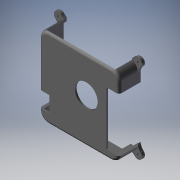
# Autodesk Inventor part: BP004
Saved by Autodesk Inventor 2017 SP1 (Build 210196100, 196)
## iProperties
Created: 2018-01-04
Part Number: BP004
Material: ABS Plastic
Document SubType Name: Modeling
Designer: Zach
Density: 1.06 g/cm^3
Appearance: CR White
Author: Zach
Autodesk Inventor part; units mm, degrees
ref_plane "YZ Plane" through (0, 0, 0) normal (1, 0, 0) x (0, 1, 0)
ref_plane "XZ Plane" through (0, 0, 0) normal (0, 1, 0) x (-1, 0, 0)
ref_plane "XY Plane" through (0, 0, 0) normal (0, 0, 1) x (1, 0, 0)
sketch "Sketch1" plane through (0, 0, 0) normal (0, 0, 1) x (1, 0, 0)
  line L0 (0, 0) -> (140, 0)
  line L1 (140, 0) -> (140, 140)
  line L2 (140, 140) -> (0, 140)
  line L3 (0, 140) -> (0, 0)
  line L4 (5, 135) -> (135, 135)
  line L5 (135, 135) -> (135, 5)
  line L6 (135, 5) -> (5, 5)
  line L7 (5, 5) -> (5, 135)
  point P0 (70, 135)
  point P1 (70, 140)
  point P2 (135, 70)
  point P3 (140, 70)
  dimension "d0" = 140
  dimension "d1" = 140
  dimension "d2" = 130
  dimension "d3" = 130
  constraints: 16 end point, 4 midpoint, 4 parallel, 2 horizontal, 2 perpendicular, 1 horizontal alignment, 1 vertical alignment
  measures "d0" distance of L2.end L1.end
  measures "d1" distance of L1.end L0.end
  measures "d2" distance of L5.end L6.end
  measures "d3" distance of L4.end L5.end
extrude "Extrusion1" add sketch "Sketch1" along normal blind 35
sketch "Sketch2" plane through (0, 0, 35) normal (0, 0, 1) x (1, 0, 0)
  line L0 (135, 5) -> (5, 5) projected
  line L1 (135, 135) -> (135, 5) projected
  line L2 (135, 5) -> (5, 5) projected
  line L3 (5, 5) -> (5, 135) projected
  line L4 (5, 135) -> (135, 135) projected
  line L5 (0, 0) -> (140, 0) projected
  line L6 (140, 0) -> (140, 140) projected
  line L7 (140, 140) -> (0, 140) projected
  line L8 (0, 140) -> (0, 0) projected
extrude "Extrusion2" add sketch "Sketch2" along normal blind 3 contours L0 L3 L4 L1 | L8 L7 L6 L5
sketch "Sketch3" plane through (0, 0, 0) normal (0, 0, -1) x (-1, 0, 0)
  line L0 (0, 0) -> (-140, 0) construction
  circle A0 centre (0, 0) radius 7.5 construction
  line L1 (0, 140) -> (0, 0) construction
  arc A1 (-7.5, 0) -> (0, 7.5) centre (0, 0) ccw
  line L2 (0, 7.5) -> (0, 0)
  line L3 (0, 0) -> (-7.5, 0)
  line L4 (-140, 140) -> (0, 140) construction
  line L5 (-140, 0) -> (-140, 140) construction
  line L6 (-70, 140) -> (-70, 0)
  line L7 (-140, 70) -> (0, 70)
  circle A2 centre (0, 140) radius 7.5 construction
  arc A3 (0, 132.5) -> (-7.5, 140) centre (0, 140) ccw
  line L8 (-7.5, 140) -> (0, 140)
  line L9 (0, 140) -> (0, 132.5)
  circle A4 centre (-140, 140) radius 7.5 construction
  arc A5 (-132.5, 140) -> (-140, 132.5) centre (-140, 140) ccw
  line L10 (-140, 132.5) -> (-140, 140)
  line L11 (-140, 140) -> (-132.5, 140)
  circle A6 centre (-140, 0) radius 7.5 construction
  arc A7 (-140, 7.5) -> (-132.5, 0) centre (-140, 0) ccw
  line L12 (-132.5, 0) -> (-140, 0)
  line L13 (-140, 0) -> (-140, 7.5)
  point P0 (-70, 70)
  dimension "d8" = 15
  dimension "d11" = 360
  constraints: 20 end point, 16 point on circle, 8 centre point, 5 concentric, 5 midpoint, 2 point on line, 1 coincident, 1 perpendicular, 1 vertical, 33 other
  measures "d8" diameter of A0
extrude "Extrusion3" add sketch "Sketch3" against normal blind 5
sketch "Sketch4" plane through (0, 0, 5) normal (0, 0, 1) x (1, 0, 0)
  line L0 (0, 0) -> (140, 0) projected
  circle A0 centre (0, 0) radius 1.5
  line L1 (140, 140) -> (0, 140) projected
  circle A1 centre (0, 140) radius 1.5
  circle A2 centre (140, 140) radius 1.5
  line L2 (140, 0) -> (140, 7.5) projected
  circle A3 centre (140, 0) radius 1.5
  dimension "d15" = 3
  dimension "d16" = 3
  dimension "d17" = 3
  dimension "d18" = 3
  constraints: 4 centre point, 3 coincident
  measures "d15" diameter of A0
  measures "d16" diameter of A1
  measures "d17" diameter of A2
  measures "d18" diameter of A3
extrude "Extrusion4" cut sketch "Sketch4" along normal through all both and the other way through all
sketch "Sketch5" plane through (0, 0, 5) normal (0, 0, 1) x (1, 0, 0)
  arc A0 (0, 1.5) -> (1.5, 0) centre (0, 0) ccw projected
  circle A1 centre (0, 0) radius 3.5
  circle A2 centre (140, 0) radius 3.5
  circle A3 centre (140, 140) radius 3.5
  circle A4 centre (0, 140) radius 3.5
  arc A5 (140, 138.5) -> (138.5, 140) centre (140, 140) ccw projected
  arc A6 (1.5, 140) -> (0, 138.5) centre (0, 140) ccw projected
  arc A7 (138.5, 0) -> (140, 1.5) centre (140, 0) ccw projected
  dimension "d21" = 7
  dimension "d22" = 7
  dimension "d23" = 7
  dimension "d24" = 7
  constraints: 4 centre point, 4 coincident
  measures "d21" diameter of A1
  measures "d22" diameter of A2
  measures "d23" diameter of A3
  measures "d24" diameter of A4
extrude "Extrusion5" cut sketch "Sketch5" along normal through all
fillet "Fillet1" radius 15 8 edges at (7.5, 140, 2.5) (132.5, 140, 2.5) (0, 7.5, 2.5) (0, 132.5, 2.5) (7.5, 0, 2.5) (132.5, 0, 2.5) (140, 132.5, 2.5) (140, 7.5, 2.5)
fillet "Fillet3" radius 15 8 edges at (140, 136.5, 21.5) (136.5, 140, 21.5) (3.5, 140, 21.5) (0, 136.5, 21.5) (0, 3.5, 21.5) (3.5, 0, 21.5) (140, 3.5, 21.5) (136.5, 0, 21.5)
fillet "Fillet4" radius 5 8 edges at (135.6067, 135.6065, 38) (70, 140, 38) (4.3935, 135.6067, 38) (0, 70, 38) (4.3935, 4.3933, 38) (70, 0, 38) (135.6065, 4.3933, 38) (140, 70, 38)
sketch "Sketch6" plane through (16.7705, 140, 0) normal (0, 1, 0) x (1, 0, 0)
  line L0 (113.2295, -35) -> (-6.7705, -35)
  line L1 (-6.7705, -35) -> (-6.7705, 0)
  line L2 (-6.7705, 0) -> (113.2295, 0)
  line L3 (113.2295, 0) -> (113.2295, -35)
  line L4 (106.459, 0) -> (0, 0) projected
  point P0 (-16.7705, 0)
  point P1 (53.2295, 0)
  dimension "d31" = 120
  dimension "d32" = 35
  constraints: 8 end point, 2 midpoint, 2 parallel, 1 horizontal, 1 perpendicular
  measures "d31" distance of L1.end L2.end
  measures "d32" distance of L0.end L1.end
extrude "Extrusion6" cut sketch "Sketch6" along normal mid plane 10
sketch "Sketch7" plane through (5, 5, 0) normal (0, 1, 0) x (1, 0, 0)
  line L0 (127.5, 10) -> (2.5, 10) construction
  line L1 (0, 0) -> (130, 0) projected
  line L2 (11.7705, 0) -> (118.2295, 0) projected
  line L3 (66.5, 0) -> (46.5, 0)
  line L4 (46.5, 0) -> (46.5, -20)
  line L5 (46.5, -20) -> (66.5, -20)
  line L6 (66.5, -20) -> (66.5, 0)
  line L7 (77.5, 0) -> (117.5, 0)
  line L8 (117.5, 0) -> (117.5, -15)
  line L9 (117.5, -15) -> (77.5, -15)
  line L10 (77.5, -15) -> (77.5, 0)
  point P0 (-5, 0)
  point P1 (65, 10)
  point P2 (65, 0)
  dimension "d35" = 125
  dimension "d36" = 10
  dimension "d37" = 20
  dimension "d38" = 20
  dimension "d39" = 44
  dimension "d40" = 75
  dimension "d41" = 40
  dimension "d42" = 15
  constraints: 18 end point, 4 parallel, 3 horizontal, 2 midpoint, 2 perpendicular, 2 point on line, 1 vertical alignment
  measures "d35" distance of L0.start L0.end
  measures "d36" distance between parallel lines of L0 L1
  measures "d37" distance of L5.end L4.end
  measures "d38" distance of L4.end L3.end
  measures "d39" distance from line of L0.end L4
  measures "d40" distance from line of L0.end L10
  measures "d41" distance of L8.end L9.end
  measures "d42" distance of L9.end L7.start
extrude "Extrusion7" cut sketch "Sketch7" against normal through all
sketch "Sketch8" plane through (0, 0, 38) normal (0, 0, 1) x (1, 0, 0)
  line L0 (132.5, 132.5) -> (7.5, 132.5) construction
  line L1 (7.5, 132.5) -> (7.5, 7.5) construction
  line L2 (7.5, 7.5) -> (132.5, 7.5) construction
  line L3 (132.5, 7.5) -> (132.5, 132.5) construction
  line L4 (140, 15) -> (140, 125) construction
  line L5 (125, 139.5826) -> (15, 139.5826) construction
  circle A0 centre (82.5, 77.5) radius 20
  line L6 (132.5, 107.5) -> (117.5, 107.5) construction
  line L7 (117.5, 107.5) -> (117.5, 12.5) construction
  line L8 (117.5, 12.5) -> (132.5, 12.5) construction
  line L9 (132.5, 12.5) -> (132.5, 107.5) construction
  line L10 (117.5, 107.5) -> (140, 107.5)
  line L11 (140, 107.5) -> (140, 12.5)
  line L12 (140, 12.5) -> (117.5, 12.5)
  line L13 (117.5, 12.5) -> (117.5, 107.5)
  line L14 (140, 15) -> (140, 16.7705) projected
  line L15 (7.5, 17.5) -> (17.5, 17.5) construction
  line L16 (17.5, 17.5) -> (17.5, 45.5) construction
  line L17 (17.5, 45.5) -> (7.5, 45.5) construction
  line L18 (7.5, 45.5) -> (7.5, 17.5) construction
  line L19 (17.5, 45.5) -> (0, 45.5)
  line L20 (0, 45.5) -> (0, 17.5)
  line L21 (0, 17.5) -> (17.5, 17.5)
  line L22 (17.5, 17.5) -> (17.5, 45.5)
  line L23 (0, 125) -> (0, 15) construction
  point P0 (0, 0)
  point P1 (132.5, 70)
  point P2 (140, 70)
  point P3 (70, 132.5)
  point P4 (70, 139.5826)
  point P5 (140, 15.8853)
  dimension "d45" = 125
  dimension "d46" = 125
  dimension "d47" = 40
  dimension "d48" = 55
  dimension "d49" = 75
  dimension "d52" = 25
  dimension "d53" = 95
  dimension "d54" = 15
  dimension "d55" = 10
  dimension "d57" = 28
  dimension "d58" = 10
  constraints: 40 end point, 10 parallel, 5 horizontal, 5 midpoint, 5 perpendicular, 3 horizontal alignment, 3 point on line, 2 vertical alignment, 1 centre point
  measures "d45" distance of L2.end L1.end
  measures "d46" distance of L1.end L0.end
  measures "d47" diameter of A0
  measures "d48" distance from line of L0 A0.centre
  measures "d49" distance from line of L1 A0.centre
  measures "d52" distance between parallel lines of L0 L6
  measures "d53" distance of L6.end L7.end
  measures "d54" distance of L7.end L8.end
  measures "d55" distance of L15.start L15.end
  measures "d57" distance of L15.end L16.end
  measures "d58" distance between parallel lines of L2 L15
extrude "Extrusion8" cut sketch "Sketch8" against normal through all
body "Solid1"
